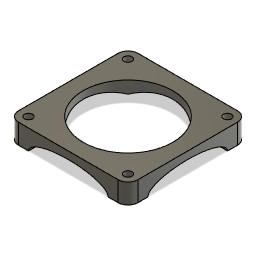
Vista_Base (Autodesk Fusion 360 design; units mm, degrees)
Autodesk Fusion 360 part; units mm, degrees
note: some values were not read from the file. Set by a fixed rule: which sketch regions a step uses.
sketch "Skizze1" plane through (0, 0, 0) normal (0, 1, 0) x (1, 0, 0)
  line L0 (10, 10) -> (-10, 10) construction
  line L1 (-10, 10) -> (-10, -10) construction
  line L2 (-10, -10) -> (10, -10) construction
  line L3 (10, -10) -> (10, 10) construction
  line L4 (10, 10) -> (-10, -10) construction
  line L5 (-10, 10) -> (10, -10) construction
  circle A0 centre (-10, 10) radius 0.8
  circle A1 centre (10, 10) radius 0.8
  circle A2 centre (10, -10) radius 0.8
  circle A3 centre (-10, -10) radius 0.8
  line L6 (12, 12) -> (-12, 12)
  line L7 (-12, 12) -> (-12, -12)
  line L8 (-12, -12) -> (12, -12)
  line L9 (12, -12) -> (12, 12)
  line L10 (12, 12) -> (-12, -12) construction
  line L11 (-12, 12) -> (12, -12) construction
  circle A4 centre (0, 0) radius 9
  dimension "d1" = 20
  dimension "d2" = 20
  dimension "d3" = 1.6
  dimension "d4" = 24
  dimension "d16" = 18
  constraint horizontal L0
  constraint perpendicular L0 L1
  constraint parallel L0 L2
  constraint parallel L1 L3
  constraint coincident L4 A4.centre
  constraint coincident L5 A4.centre
  constraint coincident A4.centre origin
  constraint coincident L0.end L1.start
  constraint coincident L0.start L3.end
  constraint coincident L2.end L3.start
  constraint coincident L1.end L2.start
  constraint equal A1 A2
  constraint equal A2 A3
  constraint equal A0 A1
  constraint horizontal L6
  constraint perpendicular L6 L7
  constraint parallel L6 L8
  constraint parallel L7 L9
  constraint coincident L10 A4.centre
  constraint coincident L11 A4.centre
  constraint collinear L4 L10
  measures "d1" distance of L1.end L2.end
  measures "d2" distance of L0.end L1.end
  measures "d3" diameter of A1
  measures "d4" distance of L6.end L7.end
  measures "d16" diameter of A4
extrude "Extrusion1" add sketch "Skizze1" along normal blind 4
sketch "Skizze2" plane through (0, 0, 12) normal (0, 0, 1) x (1, 0, 0)
  line L0 (-12, 0) -> (12, 0)
  line L1 (12, 4) -> (-12, 4)
  line L2 (-12, 4) -> (-12, 0)
  ellipse E0 centre (0, 0) end of major axis (8, 0) minor radius 2.5
  line L3 (-8, 0) -> (8, 0)
  line L4 (0, -2.5) -> (0, 2.5)
  dimension "d8" = 16
  dimension "d9" = 5
  constraint coincident E0 L3.start
  constraint coincident E0 L3.end
  constraint coincident E0 L4.start
  constraint coincident E0 L4.end
  constraint coincident E0.centre origin
  constraint parallel L0 L3
  measures "d8" distance of E0
extrude "Extrusion2" cut sketch "Skizze2" against normal blind 27 contours L0 E0 L3 L4 | L0 E0 L3 L4 picked at (-4.5024, 0.6044) picked at (4.5261, 0.5973)
sketch "Skizze3" plane through (12, 0, 0) normal (1, 0, 0) x (0, 0, -1)
  line L0 (-12, 0) -> (12, 0)
  line L1 (12, 0) -> (12, 4)
  line L2 (12, 4) -> (-12, 4)
  line L3 (-12, 4) -> (-12, 0)
  ellipse E0 centre (0, 0) end of major axis (8, 0) minor radius 2.5
  line L4 (-8, 0) -> (8, 0)
  line L5 (0, -2.5) -> (0, 2.5)
  dimension "d12" = 5
  dimension "d13" = 16
  constraint coincident E0 L4.start
  constraint coincident E0 L4.end
  constraint coincident E0 L5.start
  constraint coincident E0 L5.end
  constraint coincident E0.centre origin
  constraint parallel L0 L4
  measures "d13" distance of E0
extrude "Extrusion3" cut sketch "Skizze3" against normal blind 27 contours L0 E0 L4 L5 | L0 E0 L4 L5 picked at (-4.5024, 0.6044) picked at (4.5261, 0.5973)
fillet "Abrundung1" radius 2 4 edges at (12, 2, -12) (-12, 2, 12) (-12, 2, -12) (12, 2, 12)
equation "d1 = d2"
